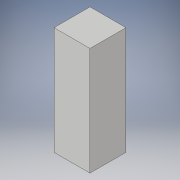
# Autodesk Inventor part: TensionerPlate
Saved by Autodesk Inventor 2017 (Build 210142000, 142)
## iProperties
Created: 2017-07-29
Part Number: TensionerPlate
Material: Generic
Document SubType Name: Modeling
Designer: User
Density: 1 g/cm^3
Appearance: Default
Author: User
Autodesk Inventor part; units mm, degrees
ref_plane "YZ Plane" through (0, 0, 0) normal (1, 0, 0) x (0, 1, 0)
ref_plane "XZ Plane" through (0, 0, 0) normal (0, 1, 0) x (-1, 0, 0)
ref_plane "XY Plane" through (0, 0, 0) normal (0, 0, 1) x (1, 0, 0)
sketch "Sketch1" plane through (0, 0, 0) normal (1, 0, 0) x (0, 1, 0)
  line L0 (31.75, 0) -> (31.75, -31.75)
  line L1 (31.75, -31.75) -> (0, -31.75)
  line L2 (0, -31.75) -> (0, 0)
  line L3 (25.4, 0) -> (25.4, -6.35)
  line L4 (25.4, -6.35) -> (6.35, -6.35)
  line L5 (6.35, -6.35) -> (6.35, 0)
  line L6 (6.35, -31.75) -> (25.4, -31.75)
  line L7 (6.35, -19.05) -> (25.4, -19.05)
  line L8 (25.4, -19.05) -> (25.4, -25.4)
  line L9 (25.4, -25.4) -> (6.35, -25.4)
  line L10 (6.35, -25.4) -> (6.35, -19.05)
  line L11 (25.4, 0) -> (6.35, 0)
  line L12 (0, 0) -> (0, 6.35)
  line L13 (0, 6.35) -> (31.75, 6.35)
  line L14 (31.75, 6.35) -> (31.75, 0)
  dimension "d6" = 6.35
  dimension "d8" = 19.05
  dimension "d9" = 6.35
  dimension "d10" = 6.35
  dimension "d11" = 6.35
  dimension "d21" = 6.35
  dimension "d22" = 31.75
  dimension "d23" = 31.75
  constraints: 30 end point, 6 parallel, 3 horizontal, 2 perpendicular, 1 point on line
  measures "d6" distance between parallel lines of L2 L5
  measures "d8" distance of L8.end L9.end
  measures "d9" distance of L7.end L8.end
  measures "d10" distance between parallel lines of L1 L9
  measures "d11" distance between parallel lines of L2 L10
  measures "d21" distance of L12.start L12.end
  measures "d22" distance of L0.start L0.end
  measures "d23" distance of L1.end L2.end
extrude "Extrusion1" add sketch "Sketch1" along normal blind 6.35 contours L3 L4 L5 L11
sketch "Sketch2" plane through (6.35, 0, 0) normal (1, 0, 0) x (0, 0, -1)
  line L0 (6.35, 25.4) -> (0, 25.4) projected
  line L1 (6.35, 6.35) -> (6.35, 25.4) projected
  line L2 (0, 6.35) -> (6.35, 6.35) projected
  circle A0 centre (12.7, 15.875) radius 4.7625
  line L3 (0, 25.4) -> (0, 6.35) projected
  point P0 (0, 0)
  dimension "d14" = 9.525
  dimension "d16" = 6.35
  constraints: 1 centre point
  measures "d14" diameter of A0
  measures "d16" distance from line of L1 A0.centre
extrude "Extrusion2" cut sketch "Sketch2" against normal blind 3.175 contours A0
equation "\"d23\" = d22"
body "Solid1"
